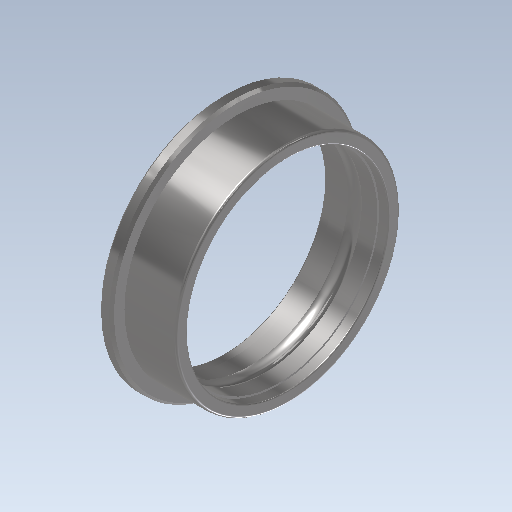
# Autodesk Inventor part: LF-1480ZZ_or
Saved by Autodesk Inventor 2021 (Build 250183000, 183)
## iProperties
Created: 2019-07-28
Part Number: LF-1480ZZ_or
Material: 鋼、炭素鋼
Catalog Web Link: www.cadenas.de
Description: Radial Flanged Ball Bearings (RF-Series/LF series) Metric ST or-Radial Flanged Ball Bearings (RF-Series/LF series) Metric Shielded Type
Vendor: NMB
Document SubType Name: Modeling
Designer: psadmin
Manufacturer: NMB
Mass: 1.24208 g
Surface Area: 4.67422 cm^2
Volume: 0.158226 cm^3
Density: 7.85 g/cm^3
Appearance: 半つや出し
Category: PARTsolutions
Company: NMB
PSOL_IDENT_0: {$CADENAS_DATA\23d-libs\nmb\pbbp\radial_flanged_ball_bearings\rfbb_rflfs_m\rflf_shielded_or.prj},223
PSOL_IDENT_1: {VTYP=3D},{NB=LF-1480ZZ_or},{LINA=LF-1480ZZ_or},{NN=Radial Flanged Ball Bearings (RF-Series/LF seri
PSOL_IDENT_2: es) Metric ST or},{DATE=11.11.2013 05:13:45},{GEOMDATE=24.10.2013 13:34:00},{VERSION=},{LINEID=1270}
PSOL_IDENT_3: ,{WBVAR=},{WBNUMERIC=}  {NB=LF-1480ZZ_or},{LINA=LF-1480ZZ_or},{KT=DUMMY},{IDNR=},{PN=LF-1480ZZ},{SHL
PSOL_IDENT_4: D=shielded},{FLANG=flanged},{SD=8.000},{D=14.000},{B=4.000},{SR=0.15},{BCZ=10},{DW=1.5875},{LI=9.90}
PSOL_IDENT_5: ,{LO=12.55},{D1=15.600},{C1=0.80},{D2=0.0},{C2=0.00},{COR=386},{CR=1036},{PCD=11.000},{U=12.588},{W=
PSOL_IDENT_6: 9.413},{Y=0.794},{Z=0.794},{AA=12.429},{AC=0.80},{AD=0.000},{AF=0.00},{AQ=0.20},{AH=12.75},{AI=10.10
PSOL_IDENT_7: },{AJ=0.40}
NN: Radial Flanged Ball Bearings (RF-Series/LF series) Metric ST or
NT: Radial Flanged Ball Bearings (RF-Series/LF series) Metric Shielded Type
NB: LF-1480ZZ_or
NBSYN: $PN._or
LINA: LF-1480ZZ_or
PN: LF-1480ZZ
SHLD: shielded
FLANG: flanged
SD: 8
D: 14
B: 4
SR: 0.15
BCZ: 10
DW: 1.5875
LI: 9.9
LO: 12.55
D1: 15.6
C1: 0.8
D2: 0
C2: 0
COR: 386
CR: 1036
PCD: 11
U: 12.588
W: 9.413
Y: 0.794
Z: 0.794
AA: 12.429
AC: 0.8
AD: 0
AF: 0
AQ: 0.2
AH: 12.75
AI: 10.1
AJ: 0.4
SUPPLIER: NMB
ARTICLENO: LF-1480ZZ_or
BOMINFO: LF-1480ZZ_or
CREATOR: CADENAS GmbH
Title: LF-1480ZZ_or
Author: Cadenas PARTsolutions
Comments: Radial Flanged Ball Bearings (RF-Series/LF series) Metric Shielded Type
Autodesk Inventor part; units mm, degrees
sketch "Sketch_3" plane through (0, 0, 0) normal (0, 0, 1) x (1, 0, 0)
  line L0 (3.85, 0) -> (0, 0)
  line L1 (0, 7.65) -> (0, 6.35)
  arc A0 (0, 6.35) -> (0.075, 6.275) centre (0.075, 6.35) ccw
  line L2 (0.075, 6.275) -> (0.605, 6.275)
  line L3 (0.605, 6.275) -> (0.605, 6.1668)
  line L4 (0.605, 6.1668) -> (1.5693, 6.1668)
  arc A1 (2.4307, 6.1668) -> (1.5693, 6.1668) centre (2, 5.5) ccw
  line L5 (2.4307, 6.1668) -> (3.4, 6.1668)
  line L6 (3.4, 6.1668) -> (3.4, 6.275)
  line L7 (3.4, 6.275) -> (3.925, 6.275)
  arc A2 (3.925, 6.275) -> (4, 6.35) centre (3.925, 6.35) ccw
  line L8 (4, 6.35) -> (4, 6.85)
  arc A3 (4, 6.85) -> (3.85, 7) centre (3.85, 6.85) ccw
  line L9 (3.85, 7) -> (0.8, 7)
  line L10 (0.8, 7) -> (0.8, 7.65)
  line L11 (0.8, 7.65) -> (0.65, 7.8)
  line L12 (0.65, 7.8) -> (0.15, 7.8)
  line L13 (0.15, 7.8) -> (0, 7.65)
  constraints: 28 end point, 8 point on circle, 4 centre point
revolve "Revolution1" add sketch "Sketch_3" angle 360 about axis through (3.85, 0, 0) along (1, 0, 0)
ref_plane "1_XY" through (2, 0, 0) normal (1, 0, 0) x (0, 0, -1)
ref_plane "1_YZ" through (2, 0, 0) normal (0, 0, -1) x (0, 1, 0)
ref_plane "1_ZX" through (2, 0, 0) normal (0, 1, 0) x (1, 0, 0)
body "Solid1"
